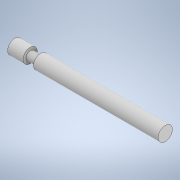
# Autodesk Inventor part: rod
Saved by Autodesk Inventor 2020 (Build 240168000, 168)
## iProperties
Created: 2021-01-29
Part Number: rod
Material: Generic
Document SubType Name: Modeling
Designer: kishore.balu
Density: 1 g/cm^3
Appearance: Default
Author: kishore.balu
Autodesk Inventor part; units mm, degrees
ref_plane "YZ Plane" through (0, 0, 0) normal (1, 0, 0) x (0, 1, 0)
ref_plane "XZ Plane" through (0, 0, 0) normal (0, 1, 0) x (-1, 0, 0)
ref_plane "XY Plane" through (0, 0, 0) normal (0, 0, 1) x (1, 0, 0)
sketch "Sketch1" plane through (0, 0, 0) normal (0, 0, 1) x (1, 0, 0)
  line L0 (0, 0) -> (0, 4.11)
  line L1 (0, 4.11) -> (9, 4.11)
  line L2 (9, 2.5) -> (9, 4.11)
  line L3 (9, 2.5) -> (15, 2.5)
  line L4 (15, 2.5) -> (15, 4.11)
  line L5 (15, 4.11) -> (87.25, 4.11)
  line L6 (0, 0) -> (87.25, 0)
  line L7 (0, 0) -> (87.25, 0)
  line L8 (87.25, 4.11) -> (87.25, 0)
  dimension "d0" = 4.11
  dimension "d1" = 9
  dimension "d3" = 6
  constraints: 18 end point, 4 perpendicular, 3 horizontal, 1 vertical
  measures "d0" distance of L0.start L0.end
  measures "d1" distance of L0.end L1.end
  measures "d3" distance of L2.start L3.end
revolve "Revolution1" add sketch "Sketch1" angle 360 about axis through (0, 0, 0) along (1, 0, 0)
body "Solid1"
